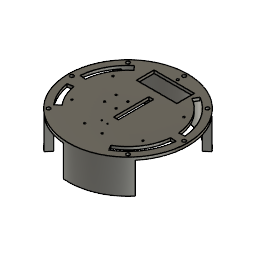
Base_Layer_Wall (Autodesk Fusion 360 design; units mm, degrees)
Autodesk Fusion 360 part; units mm, degrees
sketch "Sketch1" plane through (0, 0, 0) normal (0, 0, 1) x (1, 0, 0)
  circle A0 centre (0, 0) radius 102
  dimension "d1" = 204
  constraint coincident A0.centre origin
  measures "d1" diameter of A0
extrude "Extrude1" add sketch "Sketch1" along normal blind 5
sketch "Sketch2" plane through (0, 0, 0) normal (0, 0, -1) x (1, 0, 0)
  circle A0 centre (0, 0) radius 102
  line L0 (-68.944, -57.8509) -> (-78.1365, -65.5643)
  line L1 (0, 0) -> (102, 0) construction
  line L2 (68.944, -57.8509) -> (78.1365, -65.5643)
  line L3 (0, 0) -> (102, 0) construction
  line L4 (68.944, 57.8509) -> (78.1365, 65.5643)
  line L5 (0, 0) -> (102, 0) construction
  line L6 (-7.844, 89.6575) -> (-8.8899, 101.6119)
  line L7 (0, 0) -> (102, 0) construction
  line L8 (-68.944, 57.8509) -> (-78.1365, 65.5643)
  line L9 (0, 0) -> (102, 0) construction
  line L10 (-57.8509, 68.944) -> (-65.5643, 78.1365)
  line L11 (0, 0) -> (102, 0) construction
  arc A1 (68.944, 57.8509) -> (-7.844, 89.6575) centre (0, 0) ccw
  arc A2 (-57.8509, 68.944) -> (-68.944, 57.8509) centre (0, 0) ccw
  arc A3 (-68.944, -57.8509) -> (68.944, -57.8509) centre (0, 0) ccw
  dimension "d4" = 180
  dimension "d5" = 140
  dimension "d6" = 40
  dimension "d7" = 40
  dimension "d8" = 95
  dimension "d9" = 140
  dimension "d10" = 130
  constraint coincident A0.centre L1.start
  constraint horizontal L1
  constraint horizontal L3
  constraint horizontal L5
  constraint horizontal L7
  constraint horizontal L9
  constraint horizontal L11
  constraint concentric A1 A2
  constraint concentric A2 A3
  measures "d4" diameter of A1
  measures "d5" angle of L0 L1
  measures "d6" angle of L2 L3
  measures "d7" angle of L4 L5
  measures "d8" angle of L6 L7
  measures "d9" angle of L8 L9
  measures "d10" angle of L10 L11
extrude "Extrude2" add sketch "Sketch2" along normal blind 53 contours A0 L4 L6 A1 | A0 L0 L2 A3 | A0 L8 L10 A2
sketch "Sketch3" plane through (0, 0, -53) normal (0, 0, -1) x (1, 0, 0)
  arc A0 (-78.1365, -65.5643) -> (78.1365, -65.5643) centre (0, 0) ccw
  line L0 (78.1365, -65.5643) -> (68.944, -57.8509)
  arc A1 (-68.944, -57.8509) -> (68.944, -57.8509) centre (0, 0) ccw
  line L1 (-68.944, -57.8509) -> (-78.1365, -65.5643)
  circle A2 centre (0, 0) radius 94 construction
  line L2 (110, 0) -> (-110, 0) construction
  circle A3 centre (0, -94) radius 2.8
  line L3 (0, 0) -> (-66.468, -66.468) construction
  line L4 (0, 0) -> (94, 0) construction
  line L5 (0, 0) -> (66.468, -66.468) construction
  line L6 (0, 0) -> (94, 0) construction
  circle A4 centre (-66.468, -66.468) radius 2.8
  circle A5 centre (66.468, -66.468) radius 2.8
  circle A6 centre (66.468, 66.468) radius 2.8
  circle A7 centre (0, 94) radius 2.8
  circle A8 centre (-66.468, 66.468) radius 2.8
  dimension "d13" = 188
  dimension "d14" = 5.6
  dimension "d15" = 135
  dimension "d16" = 45
  dimension "d17" = 5.6
  dimension "d18" = 5.6
  constraint coincident A0.centre A1.centre
  constraint horizontal L2
  constraint coincident A2 A3.centre
  constraint horizontal L4
  constraint horizontal L6
  constraint coincident L3.end A4.centre
  constraint coincident L5.end A5.centre
  constraint symmetric L2 A3 A7
  constraint symmetric L2 A4 A8
  constraint symmetric L2 A5 A6
  measures "d13" diameter of A2
  measures "d14" diameter of A3
  measures "d15" angle of L3 L4
  measures "d16" angle of L5 L6
  measures "d17" diameter of A4
  measures "d18" diameter of A5
extrude "Extrude3" cut sketch "Sketch3" against normal blind 9.1 contours A3 | A4 | A5 | A6 | A7 | A8
sketch "Sketch4" plane through (0, 0, 5) normal (0, 0, 1) x (-1, 0, 0)
  circle A0 centre (0, 0) radius 102
  line L0 (0, 0) -> (0, -64) construction
  line L1 (0, 0) -> (-4.5, 0) construction
  line L2 (-4.5, 0) -> (-4.5, -5) construction
  circle A1 centre (0, 0) radius 90 construction
  circle A2 centre (0, 0) radius 96 construction
  line L3 (34.5, -79) -> (-34.5, -79)
  line L4 (-34.5, -79) -> (-34.5, -49)
  line L5 (-34.5, -49) -> (34.5, -49)
  line L6 (34.5, -49) -> (34.5, -79)
  line L7 (34.5, -79) -> (-34.5, -49) construction
  line L8 (-34.5, -79) -> (34.5, -49) construction
  line L9 (-0.5, -35) -> (-8.5, -35)
  line L10 (-8.5, -35) -> (-8.5, 25)
  line L11 (-8.5, 25) -> (-0.5, 25)
  line L12 (-0.5, 25) -> (-0.5, -35)
  line L13 (-0.5, -35) -> (-8.5, 25) construction
  line L14 (-8.5, -35) -> (-0.5, 25) construction
  line L15 (125, 0) -> (-125, 0) construction
  line L16 (0, 0) -> (-67.8823, -67.8823) construction
  line L17 (0, 0) -> (96, 0) construction
  line L18 (0, 0) -> (67.8823, -67.8823) construction
  line L19 (0, 0) -> (96, 0) construction
  circle A3 centre (67.8823, -67.8823) radius 3
  circle A4 centre (-67.8823, -67.8823) radius 3
  circle A5 centre (0, -96) radius 3
  circle A6 centre (96, 0) radius 3
  circle A7 centre (-96, 0) radius 3
  circle A8 centre (96, 0) radius 3
  circle A9 centre (67.8823, 67.8823) radius 3
  circle A10 centre (-67.8823, 67.8823) radius 3
  circle A11 centre (-96, 0) radius 3
  point P0 (0, -64)
  point P1 (-4.5, -5)
  point P2 (96, 0)
  dimension "d21" = 64
  dimension "d22" = 4.5
  dimension "d23" = 5
  dimension "d24" = 180
  dimension "d25" = 192
  dimension "d26" = 69
  dimension "d27" = 30
  dimension "d28" = 8
  dimension "d29" = 60
  dimension "d30" = 135
  dimension "d31" = 45
  dimension "d32" = 6
  dimension "d33" = 6
  dimension "d34" = 6
  dimension "d35" = 6
  dimension "d36" = 6
  constraint coincident A0.centre L0.start
  constraint vertical L0
  constraint perpendicular L0 L1
  constraint perpendicular L1 L2
  constraint horizontal L3
  constraint perpendicular L3 L4
  constraint parallel L3 L5
  constraint parallel L4 L6
  constraint coincident L7 P0
  constraint coincident L8 P0
  constraint coincident P0 L0.end
  constraint horizontal L9
  constraint perpendicular L9 L10
  constraint parallel L9 L11
  constraint parallel L10 L12
  constraint coincident L13 P1
  constraint coincident L14 P1
  constraint coincident P1 L2.end
  constraint horizontal L15
  constraint horizontal L17
  constraint horizontal L19
  constraint coincident L18.end A3.centre
  constraint coincident L16.end A4.centre
  constraint coincident A2 A5.centre
  constraint coincident P2 L17.end
  constraint coincident L15 A7.centre
  constraint coincident A2 A7.centre
  constraint symmetric L15 P2 L17.end
  constraint symmetric L15 A3 A9
  constraint symmetric L15 A4 A10
  constraint symmetric L15 A6 A8
  constraint symmetric L15 A7 A11
  measures "d21" distance of A0.centre P0
  measures "d22" distance of A0.centre L1.end
  measures "d23" distance of L1.end P1
  measures "d24" diameter of A1
  measures "d25" diameter of A2
  measures "d26" distance of L4.end L5.end
  measures "d27" distance of L3.end L4.end
  measures "d28" distance of L10.end L11.end
  measures "d29" distance of L9.end L10.end
  measures "d30" angle of L16 L17
  measures "d31" angle of L18 L19
  measures "d32" diameter of A3
  measures "d33" diameter of A4
  measures "d34" diameter of A5
  measures "d35" diameter of A6
  measures "d36" diameter of A7
extrude "Extrude4" cut sketch "Sketch4" against normal blind 10 contours L3 L4 L5 L6 | L9 L10 L11 L12 | A3 | A4 | A5 | A6 A8 | A7 A11 | A9 | A10
sketch "Sketch5" plane through (0, 0, 5) normal (0, 0, 1) x (-1, 0, 0)
  circle A0 centre (-67.8823, -67.8823) radius 3
  circle A1 centre (96, 0) radius 3
  line L0 (-34.5, -79) -> (-34.5, -49)
  line L1 (-34.5, -49) -> (34.5, -49)
  line L2 (34.5, -49) -> (34.5, -79)
  line L3 (34.5, -79) -> (-34.5, -79)
  circle A2 centre (0, -96) radius 3
  circle A3 centre (-96, 0) radius 3
  circle A4 centre (67.8823, 67.8823) radius 3
  line L4 (-8.5, -35) -> (-8.5, 25)
  line L5 (-8.5, 25) -> (-0.5, 25)
  line L6 (-0.5, 25) -> (-0.5, -35)
  line L7 (-0.5, -35) -> (-8.5, -35)
  circle A5 centre (67.8823, -67.8823) radius 3
  circle A6 centre (-67.8823, 67.8823) radius 3
  circle A7 centre (0, 0) radius 102
  circle A8 centre (0, 0) radius 90
  circle A9 centre (0, 0) radius 80
  circle A10 centre (0, 0) radius 85 construction
  circle A11 centre (85, 0) radius 2
  circle A12 centre (0, -85) radius 2
  circle A13 centre (-85, 0) radius 2
  line L8 (0, 0) -> (90, 0) construction
  line L9 (0, 0) -> (90, 0) construction
  line L10 (0, 0) -> (90, 0) construction
  line L11 (0, 0) -> (90, 0) construction
  line L12 (0, 0) -> (0, 59) construction
  line L13 (27.5, 51.5) -> (-27.5, 51.5) construction
  line L14 (-27.5, 51.5) -> (-27.5, 66.5) construction
  line L15 (-27.5, 66.5) -> (27.5, 66.5) construction
  line L16 (27.5, 66.5) -> (27.5, 51.5) construction
  line L17 (27.5, 51.5) -> (-27.5, 66.5) construction
  line L18 (-27.5, 51.5) -> (27.5, 66.5) construction
  line L19 (0, 59) -> (-15, 59) construction
  line L20 (0, 59) -> (15, 59) construction
  circle A14 centre (-15, 59) radius 1.5
  circle A15 centre (15, 59) radius 1.5
  line L21 (0, 0) -> (15, 0) construction
  line L22 (27.5, -12.5) -> (2.5, -12.5) construction
  line L23 (2.5, -12.5) -> (2.5, 12.5) construction
  line L24 (2.5, 12.5) -> (27.5, 12.5) construction
  line L25 (27.5, 12.5) -> (27.5, -12.5) construction
  line L26 (27.5, -12.5) -> (2.5, 12.5) construction
  line L27 (2.5, -12.5) -> (27.5, 12.5) construction
  circle A16 centre (27.5, -12.5) radius 1.5
  circle A17 centre (2.5, -12.5) radius 1.5
  circle A18 centre (27.5, 12.5) radius 1.5
  circle A19 centre (2.5, 12.5) radius 1.5
  line L28 (0, 0) -> (90, 0) construction
  line L29 (0, 0) -> (10.4887, -12.5)
  line L30 (51.423, -61.2836) -> (57.8509, -68.944)
  line L31 (79.6927, -7.005) -> (89.6543, -7.8806)
  line L32 (78.7846, 13.8919) -> (88.6327, 15.6283)
  line L33 (61.2836, 51.423) -> (68.944, 57.8509)
  line L34 (0, 0) -> (-0.5, -0.866)
  line L35 (-40, -69.282) -> (-45, -77.9423)
  line L36 (0, 0) -> (-0.5, -0.0437)
  line L37 (-79.6956, -6.9725) -> (-89.6575, -7.844)
  line L38 (0, 0) -> (2.5, -0.2197)
  line L39 (0, 0) -> (90, 0) construction
  line L40 (0, 0) -> (-0.5, 0.866)
  line L41 (-40, 69.282) -> (-45, 77.9423)
  line L42 (0, 0) -> (-0.5, 0.0437)
  line L43 (-79.6956, 6.9725) -> (-89.6575, 7.844)
  point P0 (0, 59)
  point P1 (15, 0)
  dimension "d39" = 180
  dimension "d40" = 160
  dimension "d41" = 170
  dimension "d42" = 4
  dimension "d43" = 4
  dimension "d44" = 4
  dimension "d45" = 50
  dimension "d46" = 175
  dimension "d47" = 120
  dimension "d49" = 59
  dimension "d50" = 55
  dimension "d51" = 15
  dimension "d52" = 15
  dimension "d53" = 15
  dimension "d54" = 3
  dimension "d55" = 3
  dimension "d56" = 15
  dimension "d57" = 25
  dimension "d58" = 25
  dimension "d59" = 3
  dimension "d60" = 3
  dimension "d61" = 3
  dimension "d62" = 3
  dimension "d64" = 175
  dimension "d65" = 125
  constraint concentric A7 A8
  constraint concentric A7 A9
  constraint concentric A7 A10
  constraint coincident A10 A11.centre
  constraint coincident A10 A12.centre
  constraint coincident A10 A13.centre
  constraint horizontal L8
  constraint coincident A7.centre A8.centre
  constraint coincident A8 L31.end
  constraint horizontal L9
  constraint horizontal L10
  constraint horizontal L11
  constraint perpendicular L9 L12
  constraint horizontal L13
  constraint perpendicular L13 L14
  constraint parallel L13 L15
  constraint parallel L14 L16
  constraint coincident L17 P0
  constraint coincident L18 P0
  constraint coincident P0 L12.end
  constraint perpendicular L12 L19
  constraint parallel L19 L20
  constraint coincident L19.end A14.centre
  constraint coincident L20.end A15.centre
  constraint parallel L8 L21
  constraint horizontal L22
  constraint perpendicular L22 L23
  constraint parallel L22 L24
  constraint parallel L23 L25
  constraint coincident L26 P1
  constraint coincident L27 P1
  constraint coincident P1 L21.end
  constraint coincident L22.start L25.end
  constraint coincident L22.end L23.start
  constraint coincident L24.end L25.start
  constraint coincident L23.end L24.start
  constraint horizontal L28
  constraint coincident L22 L29.end
  constraint coincident A9 L30.start
  constraint collinear L29 L30
  constraint coincident A9 L31.start
  constraint coincident A9 L32.start
  constraint coincident A9 L33.start
  constraint coincident A9 L35.start
  constraint coincident A9 L37.start
  constraint collinear L36 L37
  constraint coincident L6 L36.end
  constraint coincident L23 L38.end
  constraint coincident L6 L34.end
  constraint horizontal L39
  constraint coincident A9 L41.start
  constraint collinear L40 L41
  constraint coincident L6 L40.end
  constraint coincident A9 L43.start
  constraint collinear L42 L43
  constraint coincident L6 L42.end
  measures "d39" diameter of A8
  measures "d40" diameter of A9
  measures "d41" diameter of A10
  measures "d42" diameter of A11
  measures "d43" diameter of A12
  measures "d44" diameter of A13
  measures "d45" angle of L8 L29
  measures "d46" angle of L9 L36
  measures "d47" angle of L10 L34
  measures "d49" distance of A7.centre P0
  measures "d50" distance of L14.end L15.end
  measures "d51" distance of L13.end L14.end
  measures "d52" distance of P0 L19.end
  measures "d53" distance of P0 L20.end
  measures "d54" diameter of A14
  measures "d55" diameter of A15
  measures "d56" distance of A7.centre P1
  measures "d57" distance of L23.end L24.end
  measures "d58" distance of L22.end L23.end
  measures "d59" diameter of A16
  measures "d60" diameter of A17
  measures "d61" diameter of A18
  measures "d62" diameter of A19
  measures "d64" angle of L39 L42
  measures "d65" angle of L40 L42
extrude "Extrude5" cut sketch "Sketch5" against normal blind 5 contours A8 A9 L35 L37 | A8 A9 L41 L43 | A8 A9 L30 L31 | A8 A9 L32 L33 | A11 | A12 | A13 | A14 | A15
sketch "Sketch6" plane through (0, 0, 5) normal (0, 0, 1) x (-1, 0, 0)
  circle A0 centre (0, -85) radius 2
  arc A1 (-45, 77.9423) -> (-89.6575, 7.844) centre (0, 0) ccw
  line L0 (-45, 77.9423) -> (-40, 69.282)
  arc A2 (-40, 69.282) -> (-79.6956, 6.9725) centre (0, 0) ccw
  line L1 (-79.6956, 6.9725) -> (-89.6575, 7.844)
  arc A3 (88.6327, 15.6283) -> (68.944, 57.8509) centre (0, 0) ccw
  line L2 (88.6327, 15.6283) -> (78.7846, 13.8919)
  arc A4 (78.7846, 13.8919) -> (61.2836, 51.423) centre (0, 0) ccw
  line L3 (61.2836, 51.423) -> (68.944, 57.8509)
  circle A5 centre (-85, 0) radius 2
  circle A6 centre (15, 59) radius 1.5
  line L4 (-89.6575, -7.844) -> (-79.6956, -6.9725)
  arc A7 (-79.6956, -6.9725) -> (-40, -69.282) centre (0, 0) ccw
  line L5 (-40, -69.282) -> (-45, -77.9423)
  arc A8 (-89.6575, -7.844) -> (-45, -77.9423) centre (0, 0) ccw
  arc A9 (57.8509, -68.944) -> (89.6543, -7.8806) centre (0, 0) ccw
  line L6 (57.8509, -68.944) -> (51.423, -61.2836)
  arc A10 (51.423, -61.2836) -> (79.6927, -7.005) centre (0, 0) ccw
  line L7 (79.6927, -7.005) -> (89.6543, -7.8806)
  circle A11 centre (85, 0) radius 2
  circle A12 centre (-15, 59) radius 1.5
  circle A13 centre (-67.8823, -67.8823) radius 3
  circle A14 centre (96, 0) radius 3
  line L8 (-34.5, -79) -> (-34.5, -49)
  line L9 (-34.5, -49) -> (34.5, -49)
  line L10 (34.5, -49) -> (34.5, -79)
  line L11 (34.5, -79) -> (-34.5, -79)
  circle A15 centre (0, -96) radius 3
  circle A16 centre (-96, 0) radius 3
  circle A17 centre (67.8823, 67.8823) radius 3
  line L12 (-8.5, -35) -> (-8.5, 25)
  line L13 (-8.5, 25) -> (-0.5, 25)
  line L14 (-0.5, 25) -> (-0.5, -35)
  line L15 (-0.5, -35) -> (-8.5, -35)
  circle A18 centre (67.8823, -67.8823) radius 3
  circle A19 centre (-67.8823, 67.8823) radius 3
  circle A20 centre (0, 0) radius 102
  line L16 (0, 0) -> (20, 0)
  line L17 (32.5, -12.5) -> (7.5, -12.5) construction
  line L18 (7.5, -12.5) -> (7.5, 12.5) construction
  line L19 (7.5, 12.5) -> (32.5, 12.5) construction
  line L20 (32.5, 12.5) -> (32.5, -12.5) construction
  line L21 (32.5, -12.5) -> (7.5, 12.5) construction
  line L22 (7.5, -12.5) -> (32.5, 12.5) construction
  line L23 (42, 0) -> (-20, 0) construction
  line L24 (32.5, -12.5) -> (30, -12.5) construction
  line L25 (30, -12.5) -> (30, -10) construction
  line L26 (7.5, -12.5) -> (10, -12.5) construction
  line L27 (10, -12.5) -> (10, -10) construction
  circle A21 centre (30, -10) radius 1.5
  circle A22 centre (10, -10) radius 1.5
  circle A23 centre (30, 10) radius 1.5
  circle A24 centre (10, 10) radius 1.5
  point P0 (20, 0)
  dimension "d68" = 20
  dimension "d69" = 25
  dimension "d70" = 25
  dimension "d71" = 2.5
  dimension "d72" = 2.5
  dimension "d73" = 2.5
  dimension "d74" = 2.5
  dimension "d75" = 3
  dimension "d76" = 3
  constraint coincident A1.centre A2.centre
  constraint perpendicular L14 L16
  constraint horizontal L17
  constraint perpendicular L17 L18
  constraint parallel L17 L19
  constraint parallel L18 L20
  constraint coincident L21 P0
  constraint coincident L22 P0
  constraint coincident P0 L16.end
  constraint horizontal L23
  constraint perpendicular L20 L24
  constraint perpendicular L17 L25
  constraint perpendicular L18 L26
  constraint perpendicular L26 L27
  constraint coincident L25.end A21.centre
  constraint coincident L27.end A22.centre
  constraint symmetric L23 A21 A23
  constraint symmetric L23 A22 A24
  measures "d68" distance of A1.centre P0
  measures "d69" distance of L18.end L19.end
  measures "d70" distance of L17.end L18.end
  measures "d71" distance of L17.start L24.end
  measures "d72" distance of L24.end L25.end
  measures "d73" distance of L17.end L26.end
  measures "d74" distance of L26.end L27.end
  measures "d75" diameter of A21
  measures "d76" diameter of A22
extrude "Extrude6" cut sketch "Sketch6" against normal blind 5 contours A21 | A22 | A23 | A24
sketch "Sketch7" plane through (0, 0, -53) normal (0, 0, -1) x (1, 0, 0)
  circle A0 centre (66.468, -66.468) radius 2.8
  circle A1 centre (0, -94) radius 2.8
  circle A2 centre (-66.468, -66.468) radius 2.8
  arc A3 (-78.1365, -65.5643) -> (78.1365, -65.5643) centre (0, 0) ccw
  line L0 (78.1365, -65.5643) -> (68.944, -57.8509)
  arc A4 (-68.944, -57.8509) -> (68.944, -57.8509) centre (0, 0) ccw
  line L1 (-68.944, -57.8509) -> (-78.1365, -65.5643)
  line L2 (-57.8509, -68.944) -> (-65.5643, -78.1365)
  line L3 (0, 0) -> (102, 0) construction
  line L4 (-45, -77.9423) -> (-51, -88.3346)
  line L5 (0, 0) -> (102, 0) construction
  line L6 (57.8509, -68.944) -> (65.5643, -78.1365)
  line L7 (0, 0) -> (102, 0) construction
  line L8 (45, -77.9423) -> (51, -88.3346)
  line L9 (0, 0) -> (102, 0) construction
  dimension "d79" = 130
  dimension "d80" = 120
  dimension "d81" = 50
  dimension "d82" = 60
  constraint horizontal L3
  constraint coincident A3.centre A4.centre
  constraint horizontal L5
  constraint horizontal L7
  constraint horizontal L9
  constraint coincident A4 L6.start
  constraint coincident A4 L8.start
  constraint coincident A4 L4.start
  constraint coincident A4 L2.start
  measures "d79" angle of L2 L3
  measures "d80" angle of L4 L5
  measures "d81" angle of L6 L7
  measures "d82" angle of L8 L9
extrude "Extrude7" cut sketch "Sketch7" against normal blind 3 contours A3 A4 L2 L4 | A3 A4 L6 L8
sketch "Sketch8" plane through (0, 0, 5) normal (0, 0, 1) x (-1, 0, 0)
  line L0 (0, 0) -> (0, 40) construction
  line L1 (10, 32.5) -> (-10, 32.5) construction
  line L2 (-10, 32.5) -> (-10, 47.5) construction
  line L3 (-10, 47.5) -> (10, 47.5) construction
  line L4 (10, 47.5) -> (10, 32.5) construction
  line L5 (10, 32.5) -> (-10, 47.5) construction
  line L6 (-10, 32.5) -> (10, 47.5) construction
  line L7 (0, 40) -> (-5, 40) construction
  line L8 (0, 40) -> (5, 40) construction
  circle A0 centre (-5, 40) radius 1
  circle A1 centre (5, 40) radius 1
  point P0 (0, 40)
  dimension "d85" = 20
  dimension "d86" = 15
  dimension "d87" = 5
  dimension "d88" = 5
  dimension "d89" = 2
  dimension "d90" = 2
  constraint coincident L0.start origin
  constraint vertical L0
  constraint horizontal L1
  constraint perpendicular L1 L2
  constraint parallel L1 L3
  constraint parallel L2 L4
  constraint coincident L5 P0
  constraint coincident L6 P0
  constraint coincident P0 L0.end
  constraint perpendicular L0 L7
  constraint parallel L7 L8
  constraint coincident L7.end A0.centre
  constraint coincident L8.end A1.centre
  measures "d85" distance of L2.end L3.end
  measures "d86" distance of L1.end L2.end
  measures "d87" distance of P0 L7.end
  measures "d88" distance of P0 L8.end
  measures "d89" diameter of A0
  measures "d90" diameter of A1
extrude "Extrude8" cut sketch "Sketch8" against normal blind 5
sketch "Sketch9" plane through (0, 0, 5) normal (0, 0, 1) x (-1, 0, 0)
  circle A0 centre (-5, 40) radius 1
  circle A1 centre (5, 40) radius 1
  circle A2 centre (10, -10) radius 1.5
  circle A3 centre (10, 10) radius 1.5
  circle A4 centre (30, -10) radius 1.5
  circle A5 centre (30, 10) radius 1.5
  circle A6 centre (0, -85) radius 2
  arc A7 (-45, 77.9423) -> (-89.6575, 7.844) centre (0, 0) ccw
  line L0 (-45, 77.9423) -> (-40, 69.282)
  arc A8 (-40, 69.282) -> (-79.6956, 6.9725) centre (0, 0) ccw
  line L1 (-79.6956, 6.9725) -> (-89.6575, 7.844)
  arc A9 (88.6327, 15.6283) -> (68.944, 57.8509) centre (0, 0) ccw
  line L2 (88.6327, 15.6283) -> (78.7846, 13.8919)
  arc A10 (78.7846, 13.8919) -> (61.2836, 51.423) centre (0, 0) ccw
  line L3 (61.2836, 51.423) -> (68.944, 57.8509)
  circle A11 centre (-85, 0) radius 2
  circle A12 centre (15, 59) radius 1.5
  line L4 (-89.6575, -7.844) -> (-79.6956, -6.9725)
  arc A13 (-79.6956, -6.9725) -> (-40, -69.282) centre (0, 0) ccw
  line L5 (-40, -69.282) -> (-45, -77.9423)
  arc A14 (-89.6575, -7.844) -> (-45, -77.9423) centre (0, 0) ccw
  arc A15 (57.8509, -68.944) -> (89.6543, -7.8806) centre (0, 0) ccw
  line L6 (57.8509, -68.944) -> (51.423, -61.2836)
  arc A16 (51.423, -61.2836) -> (79.6927, -7.005) centre (0, 0) ccw
  line L7 (79.6927, -7.005) -> (89.6543, -7.8806)
  circle A17 centre (85, 0) radius 2
  circle A18 centre (-15, 59) radius 1.5
  circle A19 centre (-67.8823, -67.8823) radius 3
  circle A20 centre (96, 0) radius 3
  line L8 (-34.5, -79) -> (-34.5, -49)
  line L9 (-34.5, -49) -> (34.5, -49)
  line L10 (34.5, -49) -> (34.5, -79)
  line L11 (34.5, -79) -> (-34.5, -79)
  circle A21 centre (0, -96) radius 3
  circle A22 centre (-96, 0) radius 3
  circle A23 centre (67.8823, 67.8823) radius 3
  line L12 (-8.5, -35) -> (-8.5, 25)
  line L13 (-8.5, 25) -> (-0.5, 25)
  line L14 (-0.5, 25) -> (-0.5, -35)
  line L15 (-0.5, -35) -> (-8.5, -35)
  circle A24 centre (67.8823, -67.8823) radius 3
  circle A25 centre (-67.8823, 67.8823) radius 3
  circle A26 centre (0, 0) radius 102
  line L16 (125, 0) -> (-125, 0) construction
  line L17 (0, -110) -> (0, 110) construction
  circle A27 centre (0, 0) radius 70
  line L18 (0, 0) -> (60.6218, -35) construction
  line L19 (0, 0) -> (70, 0) construction
  line L20 (0, 0) -> (60.6218, 35) construction
  line L21 (0, 0) -> (70, 0) construction
  line L22 (0, 0) -> (-60.6218, -35) construction
  line L23 (0, 0) -> (70, 0) construction
  line L24 (0, 0) -> (-60.6218, 35) construction
  line L25 (0, 0) -> (70, 0) construction
  circle A28 centre (60.6218, -35) radius 1.5
  circle A29 centre (60.6218, 35) radius 1.5
  circle A30 centre (-60.6218, -35) radius 1.5
  circle A31 centre (-60.6218, 35) radius 1.5
  dimension "d93" = 140
  dimension "d94" = 30
  dimension "d95" = 30
  dimension "d96" = 150
  dimension "d97" = 150
  dimension "d98" = 3
  dimension "d99" = 3
  dimension "d100" = 3
  dimension "d101" = 3
  constraint horizontal L16
  constraint perpendicular L16 L17
  constraint concentric A7 A27
  constraint horizontal L19
  constraint coincident A7.centre A8.centre
  constraint horizontal L21
  constraint horizontal L23
  constraint horizontal L25
  constraint coincident L18.end A28.centre
  constraint coincident L20.end A29.centre
  constraint coincident L22.end A30.centre
  constraint coincident L24.end A31.centre
  measures "d93" diameter of A27
  measures "d94" angle of L18 L19
  measures "d95" angle of L20 L21
  measures "d96" angle of L22 L23
  measures "d97" angle of L24 L25
  measures "d98" diameter of A28
  measures "d99" diameter of A29
  measures "d100" diameter of A30
  measures "d101" diameter of A31
extrude "Extrude9" cut sketch "Sketch9" against normal blind 5 contours A27 A30 | A27 A30 | A27 A28 | A27 A28 | A27 A31 | A27 A31 | A27 A29 | A27 A29
sketch "Sketch10" plane through (0, 0, 0) normal (-0.996195, 0.087156, 0) x (-0.087156, -0.996195, 0)
  line L0 (102, 0) -> (90, 0)
  line L1 (90, 0) -> (90, -53)
  line L2 (90, -53) -> (102, -53)
  line L3 (102, -53) -> (102, 0)
  line L4 (95, 0) -> (90, 0)
  line L5 (90, -10) -> (90, 0)
  line L6 (90, -10) -> (95, -10)
  line L7 (95, -10) -> (95, 0)
  dimension "d104" = 10
  dimension "d105" = 5
  dimension "d106" = 43
  constraint coincident L0 L4.start
  constraint coincident L0.end L1.start
  constraint coincident L1 L5.start
  constraint perpendicular L5 L6
  constraint perpendicular L4 L7
  measures "d104" distance of L4.start L6.end
  measures "d105" distance of L5.start L6.end
  measures "d106" distance of L2 L6
revolve "Revolve1" add sketch "Sketch10" angle 90 about axis through (-8.2798, -94.6385, 0) along (0.087156, 0.996195, 0) contours L0 L1 L4 L5 L6 L7
sketch "Sketch11" plane through (0, 0, 0) normal (0.766044, -0.642788, 0) x (0.642788, 0.766044, 0)
  line L0 (-90, 0) -> (-102, 0)
  line L1 (-102, 0) -> (-102, -53)
  line L2 (-102, -53) -> (-90, -53)
  line L3 (-90, -53) -> (-90, 0)
  line L4 (-90, 0) -> (-95, 0)
  line L5 (-95, 0) -> (-95, -10)
  line L6 (-95, -10) -> (-90, -10)
  line L7 (-90, 0) -> (-90, -10)
  constraint coincident L0.start L3.end
  constraint coincident L0 L4.end
  constraint perpendicular L4 L5
  constraint coincident L3 L6.end
  constraint perpendicular L3 L6
revolve "Revolve2" add sketch "Sketch11" angle 90 about axis through (-57.8509, -68.944, 0) along (-0.642788, -0.766044, 0) contours L0 L3 L4 L5 L6 L7
sketch "Sketch12" plane through (-8.2798, -94.6385, 0) normal (-0.087156, -0.996195, 0) x (0.996195, -0.087156, 0)
  line L0 (0, -10) -> (0, 0)
  line L1 (0, 0) -> (-10, 0)
  arc A0 (-10, 0) -> (0, -10) centre (0, 0) ccw
  line L2 (0, 0) -> (-4, 0)
  line L3 (-4, 0) -> (-4, -4)
  circle A1 centre (-4, -4) radius 2.9
  dimension "d109" = 4
  dimension "d110" = 4
  dimension "d111" = 5.8
  constraint coincident L0.end L1.start
  constraint perpendicular L0 L2
  constraint perpendicular L1 L3
  constraint coincident L3.end A1.centre
  measures "d109" distance of L0.end L2.end
  measures "d110" distance of L2.end L3.end
  measures "d111" diameter of A1
extrude "Extrude10" cut sketch "Sketch12" against normal blind 5 contours A1
sketch "Sketch13" plane through (-61.0648, -72.7742, 0) normal (-0.642788, -0.766044, 0) x (0.766044, -0.642788, 0)
  line L0 (0, 0) -> (0, -10)
  arc A0 (0, -10) -> (10, 0) centre (0, 0) ccw
  line L1 (10, 0) -> (0, 0)
  line L2 (0, 0) -> (4, 0)
  line L3 (4, 0) -> (4, -4)
  circle A1 centre (4, -4) radius 2.9
  dimension "d114" = 4
  dimension "d115" = 4
  dimension "d116" = 5.8
  constraint coincident L0.start A0.centre
  constraint perpendicular L0 L2
  constraint perpendicular L2 L3
  constraint coincident L3.end A1.centre
  measures "d114" distance of L0.start L2.end
  measures "d115" distance of L2.end L3.end
  measures "d116" diameter of A1
extrude "Extrude11" cut sketch "Sketch13" against normal blind 6 contours A1
sketch "Sketch14" plane through (0, 0, 0) normal (-0.642788, 0.766044, 0) x (-0.766044, -0.642788, 0)
  line L0 (102, 0) -> (90, 0)
  line L1 (90, 0) -> (90, -53)
  line L2 (90, -53) -> (102, -53)
  line L3 (102, -53) -> (102, 0)
  line L4 (90, 0) -> (95, 0)
  line L5 (95, 0) -> (95, -10)
  line L6 (95, -10) -> (90, -10)
  line L7 (90, -10) -> (90, 0)
  dimension "d119" = 5
  dimension "d120" = 10
  constraint coincident L0.end L1.start
  constraint perpendicular L1 L4
  constraint perpendicular L4 L5
  constraint coincident L1 L6.end
  constraint perpendicular L1 L6
  measures "d119" distance of L0.end L4.end
  measures "d120" distance of L4.end L5.end
revolve "Revolve3" add sketch "Sketch14" angle 90 about axis through (-68.944, -57.8509, 0) along (0.766044, 0.642788, 0) contours L0 L1 L4 L5 L6 L7
sketch "Sketch15" plane through (0, 0, 0) normal (-0.642788, -0.766044, 0) x (0.766044, -0.642788, 0)
  line L0 (-90, 0) -> (-102, 0)
  line L1 (-102, 0) -> (-102, -53)
  line L2 (-102, -53) -> (-90, -53)
  line L3 (-90, -53) -> (-90, 0)
  line L4 (-90, 0) -> (-95, 0)
  line L5 (-95, 0) -> (-95, -10)
  line L6 (-95, -10) -> (-90, -10)
  dimension "d122" = 5
  dimension "d123" = 10
  constraint coincident L0.start L3.end
  constraint perpendicular L3 L4
  constraint perpendicular L0 L5
  constraint coincident L3 L6.end
  constraint perpendicular L3 L6
  measures "d122" distance of L0.start L4.end
  measures "d123" distance of L4.end L5.end
revolve "Revolve4" add sketch "Sketch15" angle 90 about axis through (-68.944, 57.8509, 0) along (-0.766044, 0.642788, 0) contours L0 L3 L4 L5 L6
sketch "Sketch16" plane through (-72.7742, -61.0648, 0) normal (-0.766044, -0.642788, 0) x (0.642788, -0.766044, 0)
  line L0 (0, -10) -> (0, 0)
  line L1 (0, 0) -> (-10, 0)
  arc A0 (-10, 0) -> (0, -10) centre (0, 0) ccw
  line L2 (0, 0) -> (-4, 0)
  line L3 (-4, 0) -> (-4, -4)
  circle A1 centre (-4, -4) radius 2.9
  dimension "d125" = 4
  dimension "d126" = 4
  dimension "d127" = 5.8
  constraint coincident L0.end L1.start
  constraint perpendicular L0 L2
  constraint perpendicular L2 L3
  constraint coincident L3.end A1.centre
  measures "d125" distance of L0.end L2.end
  measures "d126" distance of L2.end L3.end
  measures "d127" diameter of A1
extrude "Extrude12" cut sketch "Sketch16" against normal blind 5 contours A1
sketch "Sketch17" plane through (-72.7742, 61.0648, 0) normal (-0.766044, 0.642788, 0) x (-0.642788, -0.766044, 0)
  line L0 (0, 0) -> (0, -10)
  arc A0 (0, -10) -> (10, 0) centre (0, 0) ccw
  line L1 (10, 0) -> (0, 0)
  line L2 (0, 0) -> (4, 0)
  line L3 (4, 0) -> (4, -4)
  circle A1 centre (4, -4) radius 2.9
  dimension "d130" = 4
  dimension "d131" = 4
  dimension "d132" = 5.8
  constraint coincident L0.start A0.centre
  constraint perpendicular L0 L2
  constraint perpendicular L2 L3
  constraint coincident L3.end A1.centre
  measures "d130" distance of L0.start L2.end
  measures "d131" distance of L2.end L3.end
  measures "d132" diameter of A1
extrude "Extrude13" cut sketch "Sketch17" against normal blind 5 contours A1
sketch "Sketch18" plane through (0, 0, 5) normal (0, 0, 1) x (-1, 0, 0)
  circle A0 centre (60.6218, 35) radius 1.5
  circle A1 centre (-60.6218, 35) radius 1.5
  circle A2 centre (60.6218, -35) radius 1.5
  circle A3 centre (-60.6218, -35) radius 1.5
  circle A4 centre (-5, 40) radius 1
  circle A5 centre (5, 40) radius 1
  circle A6 centre (10, -10) radius 1.5
  circle A7 centre (10, 10) radius 1.5
  circle A8 centre (30, -10) radius 1.5
  circle A9 centre (30, 10) radius 1.5
  circle A10 centre (0, -85) radius 2
  arc A11 (-45, 77.9423) -> (-89.6575, 7.844) centre (0, 0) ccw
  line L0 (-45, 77.9423) -> (-40, 69.282)
  arc A12 (-40, 69.282) -> (-79.6956, 6.9725) centre (0, 0) ccw
  line L1 (-79.6956, 6.9725) -> (-89.6575, 7.844)
  arc A13 (88.6327, 15.6283) -> (68.944, 57.8509) centre (0, 0) ccw
  line L2 (88.6327, 15.6283) -> (78.7846, 13.8919)
  arc A14 (78.7846, 13.8919) -> (61.2836, 51.423) centre (0, 0) ccw
  line L3 (61.2836, 51.423) -> (68.944, 57.8509)
  circle A15 centre (-85, 0) radius 2
  circle A16 centre (15, 59) radius 1.5
  line L4 (-89.6575, -7.844) -> (-79.6956, -6.9725)
  arc A17 (-79.6956, -6.9725) -> (-40, -69.282) centre (0, 0) ccw
  line L5 (-40, -69.282) -> (-45, -77.9423)
  arc A18 (-89.6575, -7.844) -> (-45, -77.9423) centre (0, 0) ccw
  arc A19 (57.8509, -68.944) -> (89.6543, -7.8806) centre (0, 0) ccw
  line L6 (57.8509, -68.944) -> (51.423, -61.2836)
  arc A20 (51.423, -61.2836) -> (79.6927, -7.005) centre (0, 0) ccw
  line L7 (79.6927, -7.005) -> (89.6543, -7.8806)
  circle A21 centre (85, 0) radius 2
  circle A22 centre (-15, 59) radius 1.5
  circle A23 centre (-67.8823, -67.8823) radius 3
  circle A24 centre (96, 0) radius 3
  line L8 (-34.5, -79) -> (-34.5, -49)
  line L9 (-34.5, -49) -> (34.5, -49)
  line L10 (34.5, -49) -> (34.5, -79)
  line L11 (34.5, -79) -> (-34.5, -79)
  circle A25 centre (0, -96) radius 3
  circle A26 centre (-96, 0) radius 3
  circle A27 centre (67.8823, 67.8823) radius 3
  line L12 (-8.5, -35) -> (-8.5, 25)
  line L13 (-8.5, 25) -> (-0.5, 25)
  line L14 (-0.5, 25) -> (-0.5, -35)
  line L15 (-0.5, -35) -> (-8.5, -35)
  circle A28 centre (67.8823, -67.8823) radius 3
  circle A29 centre (-67.8823, 67.8823) radius 3
  circle A30 centre (0, 0) radius 102
  circle A31 centre (-85, 0) radius 2
  circle A32 centre (85, 0) radius 2
  constraint concentric A15 A31
  constraint concentric A21 A32
extrude "Extrude14" add sketch "Sketch18" against normal blind 5 contours A15 A31 | A21 A32
